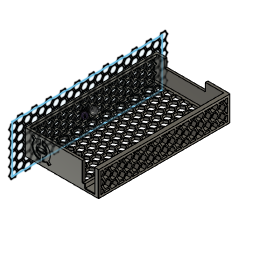
[a]BTT_MMB_case_top (Autodesk Fusion 360 design; units mm, degrees)
Autodesk Fusion 360 part; units mm, degrees
note: some values were not read from the file. Chosen so that the rebuilt part matches the saved one: which face or edge a step refers to. Set by a fixed rule: which sketch regions a step uses.
(part 1 of 3)
sketch "Top" plane through (0, 0, 0) normal (0, 0, 1) x (1, 0, 0)
  line L0 (8.6, 62.3) -> (62.6, 62.3) construction
  line L1 (62.6, 62.3) -> (62.6, -62.3) construction
  line L2 (62.6, -62.3) -> (8.6, -62.3) construction
  line L3 (8.6, -62.3) -> (8.6, 62.3) construction
  line L4 (8.6, 0) -> (0, 0) construction
  line L5 (62.8, -62.5) -> (8.4, -62.5)
  line L6 (8.4, -62.5) -> (8.4, 62.5)
  line L7 (8.4, 62.5) -> (62.8, 62.5)
  line L8 (62.8, 62.5) -> (62.8, -62.5)
  line L9 (6, -64.9) -> (6, 64.9)
  line L10 (6, 64.9) -> (65.2, 64.9)
  line L11 (65.2, 64.9) -> (65.2, -64.9)
  line L12 (65.2, -64.9) -> (6, -64.9)
  line L13 (8.6, 62.3) -> (13.6, 62.3) construction
  line L14 (13.6, 62.3) -> (13.6, 59.3) construction
  line L15 (13.6, 59.3) -> (8.6, 59.3) construction
  line L16 (8.6, 59.3) -> (8.6, 62.3) construction
  circle A0 centre (13.6, 59.3) radius 1.75
  circle A1 centre (13.6, 59.3) radius 5
  line L17 (13.6, 54.3) -> (8.4, 54.3)
  line L18 (18.6, 59.3) -> (18.6, 62.5)
  line L19 (35.6, 62.3) -> (35.6, 51.9797) construction
  circle A2 centre (57.6, 59.3) radius 5
  circle A3 centre (57.6, 59.3) radius 1.75
  line L20 (57.6, 54.3) -> (62.8, 54.3)
  line L21 (52.6, 59.3) -> (52.6, 62.5)
  line L22 (20, 0) -> (2.5, 0)
  circle A4 centre (13.6, -59.3) radius 5
  line L23 (18.6, -59.3) -> (18.6, -62.5)
  circle A5 centre (13.6, -59.3) radius 1.75
  line L24 (13.6, -54.3) -> (8.4, -54.3)
  circle A6 centre (57.6, -59.3) radius 1.75
  line L25 (57.6, -54.3) -> (62.8, -54.3)
  line L26 (52.6, -59.3) -> (52.6, -62.5)
  circle A7 centre (57.6, -59.3) radius 5
  line L27 (65.2, -64.9) -> (78.5, -64.9)
  line L28 (78.5, -64.9) -> (78.5, 64.9)
  line L29 (78.5, 64.9) -> (65.2, 64.9)
  line L30 (65.2, 64.9) -> (65.2, -64.9)
  line L31 (78.5, -64.9) -> (74.5, -64.9)
  line L32 (74.5, -64.9) -> (74.5, 64.9)
  line L33 (74.5, 64.9) -> (78.5, 64.9)
  line L34 (78.5, 64.9) -> (78.5, -64.9)
  line L35 (78.5, 64.9) -> (62.8, 64.9)
  line L36 (62.8, 64.9) -> (62.8, 62.5)
  line L37 (62.8, 62.5) -> (78.5, 62.5)
  line L38 (78.5, 62.5) -> (78.5, 64.9)
  line L39 (62.8, -62.5) -> (62.8, -64.9)
  line L40 (13.6, -54.3) -> (13.6, 54.3)
  line L41 (57.6, 54.3) -> (57.6, -54.3)
  line L42 (18.6, 62.5) -> (18.6, 64.9)
  line L43 (52.6, 62.5) -> (52.6, 64.9)
  circle A8 centre (13.6, 59.3) radius 2.95
  circle A9 centre (57.6, 59.3) radius 2.95
  circle A10 centre (57.6, -59.3) radius 2.95
  circle A11 centre (13.6, -59.3) radius 2.95
  line L44 (13.6, -54.3) -> (13.6, -62.5)
  line L45 (13.6, 54.3) -> (13.6, 62.5)
  line L46 (57.6, 54.3) -> (57.6, 62.5)
  line L47 (57.6, -54.3) -> (57.6, -62.5)
  line L48 (8.6, 60.1) -> (62.6, 60.1)
  line L49 (62.6, -60.1) -> (8.6, -60.1)
  line L50 (62.6, -60.1) -> (63.1136, -60.1)
  line L51 (8.6, -60.1) -> (8.2021, -60.1)
  line L52 (8.6, 60.1) -> (8.1648, 60.1)
  line L53 (62.6, 60.1) -> (63.3075, 60.1)
  line L54 (56.5, 64.9) -> (16.5, 64.9)
  line L55 (16.5, 64.9) -> (16.5, 54.9)
  line L56 (16.5, 54.9) -> (56.5, 54.9)
  line L57 (56.5, 54.9) -> (56.5, 64.9)
  line L58 (78.5, 64.9) -> (16.5, 64.9)
  point P0 (13.6, -59.3)
  dimension "d1" = 54
  dimension "d2" = 124.6
  dimension "d3" = 8.6
  dimension "d4" = -0.2
  dimension "d5" = -2.6
  dimension "d6" = 5
  dimension "d7" = 3
  dimension "d8" = 3.5
  dimension "d9" = 10
  dimension "d10" = 13.3
  dimension "d12" = 4
  dimension "d41" = 5.9
  dimension "d42" = 5.9
  dimension "d43" = 5.9
  dimension "d44" = 5.9
  dimension "d97" = 2.2
  dimension "d98" = 2.2
  dimension "d99" = 40
  dimension "d100" = 10
  dimension "d101" = 62
  dimension "d103" = 129.8
  constraint horizontal L0
  constraint vertical L1
  constraint horizontal L2
  constraint vertical L3
  constraint midpoint L3 L4.start
  constraint coincident L4.end origin
  constraint horizontal L4
  constraint horizontal L13
  constraint vertical L14
  constraint horizontal L15
  constraint vertical L16
  constraint coincident L14.end L15.start
  constraint concentric A0 A1
  constraint coincident A1 L17.start
  constraint coincident L6 L17.end
  constraint tangent A1 L17
  constraint perpendicular L6 L17
  constraint coincident A1 L18.start
  constraint coincident L7 L18.end
  constraint tangent A1 L18
  constraint perpendicular L7 L18
  constraint midpoint L0 L19.start
  constraint perpendicular L0 L19
  constraint symmetric A0 L19 A3
  constraint symmetric A1 L19 A2
  constraint symmetric L17.start L19 L20.start
  constraint symmetric L17.end L19 L20.end
  constraint symmetric L18.start L19 L21.start
  constraint symmetric L18.end L19 L21.end
  constraint symmetric L14.end L22 P0
  constraint symmetric A0 L22 A5
  constraint symmetric A1 L22 A4
  constraint symmetric L17.start L22 L24.start
  constraint symmetric L17.end L22 L24.end
  constraint symmetric L18.start L22 L23.start
  constraint symmetric L18.end L22 L23.end
  constraint symmetric L20.start L22 L25.start
  constraint symmetric A2 L22 A7
  constraint symmetric A3 L22 A6
  constraint symmetric L20.end L22 L25.end
  constraint symmetric L21.start L22 L26.start
  constraint symmetric L21.end L22 L26.end
  constraint horizontal L27
  constraint vertical L28
  constraint horizontal L29
  constraint vertical L30
  constraint horizontal L31
  constraint vertical L32
  constraint horizontal L33
  constraint vertical L34
  constraint coincident L29 L32.end
  constraint horizontal L35
  constraint vertical L36
  constraint horizontal L37
  constraint vertical L38
  constraint coincident L12 L39.end
  constraint perpendicular L12 L39
  constraint coincident L10 L42.end
  constraint perpendicular L10 L42
  constraint coincident L10 L43.end
  constraint perpendicular L10 L43
  constraint concentric A2 A9
  constraint concentric A6 A10
  constraint coincident P0 A4.centre
  constraint coincident L5 L44.end
  constraint perpendicular L5 L44
  constraint coincident L7 L45.end
  constraint perpendicular L7 L45
  constraint coincident L7 L46.end
  constraint perpendicular L7 L46
  constraint coincident L5 L47.end
  constraint perpendicular L5 L47
  constraint perpendicular L1 L50
  constraint perpendicular L6 L51
  constraint perpendicular L6 L52
  constraint perpendicular L8 L53
  constraint horizontal L54
  constraint vertical L55
  constraint horizontal L56
  constraint vertical L57
  constraint perpendicular L43 L58
  measures "d1" distance of L0.start L0.end
  measures "d2" distance of L0.start L2.end
  measures "d3" distance of L4.start L4.end
  measures "d6" distance of L0.start L13.end
  measures "d7" distance of L0.start L15.end
  measures "d8" diameter of A0
  measures "d9" diameter of A1
  measures "d10" distance of L11.end L27.end
  measures "d12" distance of L27.end L31.end
  measures "d41" diameter of A8
  measures "d42" diameter of A9
  measures "d43" diameter of A10
  measures "d44" diameter of A11
  measures "d99" distance of L54.start L54.end
  measures "d100" distance of L54.start L56.end
  measures "d101" distance of L28.end L54.end
  measures "d103" distance of L27.end L28.end
extrude "Extrude1" add sketch "Top" along normal blind 2.5 contours L5 L6 L9 L12 L22 A4 A7 L39 | L5 L26 A7 L49 | L5 L23 L26 L49 | L5 A4 L23 L49 | L5 A7 A10 L47 L49 | L5 A7 | L5 A4 | L5 A4 A11 L44 L49 | L5 A7 A10 L47 L49 | L5 L8 A7 L49 L50 | L5 A4 A11 L44 L49 | L5 L6 A4 L49 L51 | A6 A10 L47 L49 | A6 A10 L47 L49 | L8 L11 L12 L30 L37 L39 | A5 A11 L44 L49 | A5 A11 L44 L49 | A6 L47 L49 | A6 L47 L49 | A5 L44 L49 | A5 L44 L49 | L11 L27 L30 L32 L37 | L6 L7 L9 L10 A1 L22 L55 | L10 L11 L30 L35 L36 L37 L58 | L11 L29 L30 L32 L35 L37 L58 | L27 L28 L31 L32 L34 L37 | L7 L8 A2 L48 L53 | L7 A2 A9 L46 L48 | L6 L7 A1 L48 L52 | L7 A1 A8 L45 L48 | L7 L10 A2 L36 L57 L58 | L28 L29 L32 L33 L34 L35 L37 L38 L58 | L7 A2 L57 | A3 A9 L46 L48 | L7 A2 L21 L48 | L7 A2 A9 L48 L57 | L7 L18 L21 L48 | A3 A9 L48 L57 | A3 L46 L48 L57 | A3 L46 L48 | L7 A1 L55 | A0 A8 L45 L48 | L7 L10 A1 L42 L54 L55 L58 | L7 A9 L46 L57 | L7 A2 L57 | L7 L10 A2 L43 L54 L57 L58 | A3 A9 L46 L57 | L7 L10 L42 L43 L54 L58 | L7 A1 L18 L48 | A3 L48 L57 | L7 A8 L45 L48 L55 | L7 A1 L55 | A0 A8 L45 L48 | A0 L45 L48 | L7 A1 L48 L55 | A0 L45 L48 picked at (59.849, -60.491) picked at (55.351, -60.491) picked at (15.849, -60.491) picked at (11.351, -60.491) picked at (57.6797, -60.7279) picked at (57.5203, -60.7279) picked at (13.6797, -60.7279) picked at (13.5203, -60.7279) picked at (59.849, 60.491) picked at (55.3319, 60.4563) picked at (56.9315, 60.3325) picked at (57.6797, 60.7279) picked at (11.351, 60.491) picked at (56.8289, 61.7259) picked at (56.3305, 60.3011) picked at (15.849, 60.491) picked at (13.5203, 60.7279) picked at (13.6797, 60.7279) makes body 1
extrude "Extrude2" add sketch "Top" along normal blind 25.05 separate body contours L5 L6 L9 L12 L22 A4 A7 L39 | L5 A7 | L5 A4 | L6 L7 L9 L10 A1 L22 L55 | L10 L11 L30 L35 L36 L37 L58 | L11 L29 L30 L32 L35 L37 L58 | L27 L28 L31 L32 L34 L37 | L7 L10 A2 L36 L57 L58 | L28 L29 L32 L33 L34 L35 L37 L38 L58 | L7 A2 L57 | L7 A1 L55 picked at (57.0926, 63.094) picked at (15.3203, 62.9199) makes body 2 at (6, -21.6333, 16.7) makes body 3 at (78.5, 21.6333, 16.7)
extrude "Extrude3" add sketch "Top" along normal blind 17 contours L7 A1 L55 | L7 L10 A1 L42 L54 L55 L58 | L7 A2 L57 | L7 L10 A2 L43 L54 L57 L58 | L7 L10 L42 L43 L54 L58 | L7 A1 L55 picked at (56.2909, 63.5566) bodies 1 2 3
extrude "Extrude4" add sketch "Top" along normal blind 6.4 contours L8 L11 L12 L30 L37 L39 bodies 1
sketch "Logo?" plane through (0, 0, 0) normal (0, 1, 0) x (1, 0, 0)
  line L0 (0, 0) -> (22, 0)
  line L1 (22, -13.2) -> (22, 0) construction
  line L2 (22, -13.2) -> (22, -15) construction
  line L3 (22, -13.2) -> (22, -11.4) construction
  line L4 (19.65, -15) -> (24.35, -15)
  line L5 (19.65, -11.4) -> (24.35, -11.4)
  circle A0 centre (19.6404, -13.2) radius 1.8
  circle A1 centre (24.3416, -13.2) radius 1.8
  line L6 (22, -11.4) -> (22, -15) construction
  circle A2 centre (22, -13.2) radius 5
  circle A3 centre (22, -13.2) radius 9
  line L7 (22, -13.2) -> (28.364, -6.836) construction
  line L8 (22, -13.2) -> (31, -13.2) construction
  line L9 (22, -13.2) -> (15.636, -19.564) construction
  line L10 (22, -13.2) -> (31, -13.2) construction
  line L11 (21, -15) -> (23, -15)
  line L12 (23, -15) -> (23, -23.0446)
  line L13 (21, -15) -> (21, -23.9495)
  line L14 (21, -11.4) -> (21, -3.5444)
  line L15 (23.2543, -11.4) -> (23.2543, -2.8723)
  line L16 (14.6814, -18.3972) -> (16.8028, -20.5186)
  line L17 (14.6814, -18.3972) -> (17.9289, -18.3972) construction
  line L18 (15.636, -19.564) -> (15.7421, -19.4579)
  line L19 (14.6814, -18.3972) -> (12.5601, -20.5186)
  line L20 (16.8028, -20.5186) -> (14.6814, -22.6399)
  line L21 (22, -13.2) -> (22.0813, -13.2813)
  line L22 (22, -13.2) -> (17.5038, -8.7038) construction
  line L23 (22, -13.2) -> (28.3586, -13.2) construction
  line L24 (27.1972, -5.8814) -> (29.3186, -3.7601)
  line L25 (29.3186, -8.0028) -> (31.4399, -5.8814)
  line L26 (12.5601, -20.5186) -> (14.6814, -22.6399)
  line L27 (29.3186, -3.7601) -> (31.4399, -5.8814)
  dimension "d21" = 22
  dimension "d22" = 13.2
  dimension "d24" = 1.8
  dimension "d25" = 4.7
  dimension "d26" = 4.7
  dimension "d27" = 10
  dimension "d28" = 18
  dimension "d29" = 45
  dimension "d30" = 135
  dimension "d31" = 2
  dimension "d32" = 45
  dimension "d33" = 3
  dimension "d34" = 0.15
  dimension "d35" = 3
  dimension "d37" = 135
  constraint coincident L0.start origin
  constraint horizontal L0
  constraint perpendicular L0 L1
  constraint perpendicular L2 L4
  constraint perpendicular L1 L5
  constraint midpoint L2.end L4
  constraint midpoint L3.end L5
  constraint coincident L5.start A0
  constraint coincident L4.start A0
  constraint coincident L5.end A1
  constraint coincident L4.end A1
  constraint coincident L1.start L2.start
  constraint concentric A2 A3
  constraint horizontal L8
  constraint coincident A3 L7.end
  constraint horizontal L10
  constraint coincident A3 L9.end
  constraint perpendicular L2 L11
  constraint midpoint L2.end L11
  constraint perpendicular L4 L12
  constraint perpendicular L4 L13
  constraint coincident L5 L14.start
  constraint perpendicular L5 L14
  constraint coincident L5 L15.start
  constraint perpendicular L5 L15
  constraint vertical L13
  constraint horizontal L17
  constraint parallel L9 L18
  constraint midpoint L16 L18.end
  constraint perpendicular L16 L19
  constraint perpendicular L16 L20
  constraint perpendicular L9 L21
  constraint horizontal L23
  constraint symmetric L16.start L22 L24.start
  constraint symmetric L16.end L22 L25.start
  constraint symmetric L19.end L22 L24.end
  constraint symmetric L20.end L22 L25.end
  constraint perpendicular L20 L26
  measures "d21" distance of L0.start L0.end
  measures "d22" distance of L0.end L1.start
  measures "d24" distance of L1.start L3.end
  measures "d25" distance of L4.start L4.end
  measures "d26" distance of L5.start L5.end
  measures "d27" diameter of A2
  measures "d28" diameter of A3
  measures "d29" angle of L7 L8
  measures "d30" angle of L9 L10
  measures "d31" distance of L11.start L11.end
  measures "d32" angle of L16 L17
  measures "d33" distance of L16.start L16.end
  measures "d34" distance of L9.end L18.end
  measures "d35" distance of L16.start L19.end
  measures "d37" angle of L22 L23
extrude "Extrude5" cut sketch "Logo?" along normal blind 0.8 from surface at -64.9 contours L4 L5 A0 A1 L11 | A0 | A2 A3 L13 L14 L16 L19 L20 | A2 A3 L12 L15 | A3 L19 L20 L26 | A3 L16 L18 L20 | A3 L16 L18 L19 | A3 L24 L25 L27 bodies 1
extrude "Extrude6" [suppressed]
sketch "Top Hex" plane through (0, 0, 0) normal (0, 0, 1) x (1, 0, 0)
  line L0 (0, 0) -> (1, 0) construction
  line L1 (1, 0) -> (1, 2) construction
  line L2 (1, 2) -> (0, 2) construction
  line L3 (0, 2) -> (0, 0) construction
  line L4 (4.3758, 3.949) -> (1, 5.8981)
  line L5 (1, 5.8981) -> (-2.3758, 3.949)
  line L6 (-2.3758, 3.949) -> (-2.3758, 0.051)
  line L7 (-2.3758, 0.051) -> (1, -1.8981)
  line L8 (1, -1.8981) -> (4.3758, 0.051)
  line L9 (4.3758, 0.051) -> (4.3758, 3.949)
  line L10 (1, 2) -> (2.6879, 4.9236) construction
  line L11 (1, 2) -> (2.6879, -0.9236) construction
  line L12 (8.3546, 10.8404) -> (4.9788, 12.7895)
  line L13 (8.3546, 6.9424) -> (8.3546, 10.8404)
  line L14 (4.9788, 4.9933) -> (8.3546, 6.9424)
  line L15 (1.6029, 6.9424) -> (4.9788, 4.9933)
  line L16 (1.6029, 10.8404) -> (1.6029, 6.9424)
  line L17 (4.9788, 12.7895) -> (1.6029, 10.8404)
  line L18 (-26.5739, 91.794) -> (105.9394, 91.794)
  line L19 (105.9394, 91.794) -> (105.9394, -79.3105)
  line L20 (105.9394, -79.3105) -> (-26.5739, -79.3105)
  line L21 (-26.5739, -79.3105) -> (-26.5739, 91.794)
  line L22 (4.3758, 2) -> (5.5758, 2)
  line L23 (1.6029, -62.7776) -> (4.9788, -64.7267)
  line L24 (1.6029, -58.8796) -> (1.6029, -62.7776)
  line L25 (4.9788, -56.9305) -> (1.6029, -58.8796)
  line L26 (8.3546, -58.8796) -> (4.9788, -56.9305)
  line L27 (4.9788, -64.7267) -> (8.3546, -62.7776)
  line L28 (4.3758, -69.669) -> (4.3758, -65.771)
  line L29 (4.3758, -65.771) -> (1, -63.8219)
  line L30 (1, -63.8219) -> (-2.3758, -65.771)
  line L31 (-2.3758, -65.771) -> (-2.3758, -69.669)
  line L32 (-2.3758, -69.669) -> (1, -71.6181)
  line L33 (1, -71.6181) -> (4.3758, -69.669)
  line L34 (9.5604, -62.7776) -> (12.9363, -64.7267)
  line L35 (9.5604, -58.8796) -> (9.5604, -62.7776)
  line L36 (12.9363, -56.9305) -> (9.5604, -58.8796)
  line L37 (16.3121, -58.8796) -> (12.9363, -56.9305)
  line L38 (12.9363, -64.7267) -> (16.3121, -62.7776)
  line L39 (12.3333, -69.669) -> (12.3333, -65.771)
  line L40 (12.3333, -65.771) -> (8.9575, -63.8219)
  line L41 (8.9575, -63.8219) -> (5.5817, -65.771)
  line L42 (5.5817, -65.771) -> (5.5817, -69.669)
  line L43 (5.5817, -69.669) -> (8.9575, -71.6181)
  line L44 (8.9575, -71.6181) -> (12.3333, -69.669)
  line L45 (8.3546, -62.7776) -> (8.3546, -58.8796)
  line L46 (16.3121, -62.7776) -> (16.3121, -58.8796)
  line L47 (4.9788, 12.7895) -> (4.9788, 13.9895) construction
  line L48 (3.9166, 13.9895) -> (6.0409, 13.9895) construction
  line L49 (17.5179, -62.7776) -> (20.8938, -64.7267)
  line L50 (17.5179, -58.8796) -> (17.5179, -62.7776)
  line L51 (20.8938, -56.9305) -> (17.5179, -58.8796)
  line L52 (24.2696, -58.8796) -> (20.8938, -56.9305)
  line L53 (20.8938, -64.7267) -> (24.2696, -62.7776)
  line L54 (20.2908, -69.669) -> (20.2908, -65.771)
  line L55 (20.2908, -65.771) -> (16.915, -63.8219)
  line L56 (16.915, -63.8219) -> (13.5392, -65.771)
  line L57 (13.5392, -65.771) -> (13.5392, -69.669)
  line L58 (13.5392, -69.669) -> (16.915, -71.6181)
  line L59 (16.915, -71.6181) -> (20.2908, -69.669)
  line L60 (24.2696, -62.7776) -> (24.2696, -58.8796)
  line L61 (25.4754, -62.7776) -> (28.8513, -64.7267)
  line L62 (25.4754, -58.8796) -> (25.4754, -62.7776)
  line L63 (28.8513, -56.9305) -> (25.4754, -58.8796)
  line L64 (32.2271, -58.8796) -> (28.8513, -56.9305)
  line L65 (28.8513, -64.7267) -> (32.2271, -62.7776)
  line L66 (28.2483, -69.669) -> (28.2483, -65.771)
  line L67 (28.2483, -65.771) -> (24.8725, -63.8219)
  line L68 (24.8725, -63.8219) -> (21.4967, -65.771)
  line L69 (21.4967, -65.771) -> (21.4967, -69.669)
  line L70 (21.4967, -69.669) -> (24.8725, -71.6181)
  line L71 (24.8725, -71.6181) -> (28.2483, -69.669)
  line L72 (32.2271, -62.7776) -> (32.2271, -58.8796)
  line L73 (33.4329, -62.7776) -> (36.8088, -64.7267)
  line L74 (33.4329, -58.8796) -> (33.4329, -62.7776)
  line L75 (36.8088, -56.9305) -> (33.4329, -58.8796)
  line L76 (40.1846, -58.8796) -> (36.8088, -56.9305)
  line L77 (36.8088, -64.7267) -> (40.1846, -62.7776)
  line L78 (36.2058, -69.669) -> (36.2058, -65.771)
  line L79 (36.2058, -65.771) -> (32.83, -63.8219)
  line L80 (32.83, -63.8219) -> (29.4542, -65.771)
  line L81 (29.4542, -65.771) -> (29.4542, -69.669)
  line L82 (29.4542, -69.669) -> (32.83, -71.6181)
  line L83 (32.83, -71.6181) -> (36.2058, -69.669)
  line L84 (40.1846, -62.7776) -> (40.1846, -58.8796)
  line L85 (41.3904, -62.7776) -> (44.7663, -64.7267)
  line L86 (41.3904, -58.8796) -> (41.3904, -62.7776)
  line L87 (44.7663, -56.9305) -> (41.3904, -58.8796)
  line L88 (48.1421, -58.8796) -> (44.7663, -56.9305)
  line L89 (44.7663, -64.7267) -> (48.1421, -62.7776)
  line L90 (44.1633, -69.669) -> (44.1633, -65.771)
  line L91 (44.1633, -65.771) -> (40.7875, -63.8219)
  line L92 (40.7875, -63.8219) -> (37.4117, -65.771)
  line L93 (37.4117, -65.771) -> (37.4117, -69.669)
  line L94 (37.4117, -69.669) -> (40.7875, -71.6181)
  line L95 (40.7875, -71.6181) -> (44.1633, -69.669)
  line L96 (48.1421, -62.7776) -> (48.1421, -58.8796)
  line L97 (49.3479, -62.7776) -> (52.7238, -64.7267)
  line L98 (49.3479, -58.8796) -> (49.3479, -62.7776)
  line L99 (52.7238, -56.9305) -> (49.3479, -58.8796)
  line L100 (56.0996, -58.8796) -> (52.7238, -56.9305)
  line L101 (52.7238, -64.7267) -> (56.0996, -62.7776)
  line L102 (52.1208, -69.669) -> (52.1208, -65.771)
  line L103 (52.1208, -65.771) -> (48.745, -63.8219)
  line L104 (48.745, -63.8219) -> (45.3692, -65.771)
  line L105 (45.3692, -65.771) -> (45.3692, -69.669)
  line L106 (45.3692, -69.669) -> (48.745, -71.6181)
  line L107 (48.745, -71.6181) -> (52.1208, -69.669)
  line L108 (56.0996, -62.7776) -> (56.0996, -58.8796)
  line L109 (57.3054, -62.7776) -> (60.6813, -64.7267)
  line L110 (57.3054, -58.8796) -> (57.3054, -62.7776)
  line L111 (60.6813, -56.9305) -> (57.3054, -58.8796)
  line L112 (64.0571, -58.8796) -> (60.6813, -56.9305)
  line L113 (60.6813, -64.7267) -> (64.0571, -62.7776)
  line L114 (60.0783, -69.669) -> (60.0783, -65.771)
  line L115 (60.0783, -65.771) -> (56.7025, -63.8219)
  line L116 (56.7025, -63.8219) -> (53.3267, -65.771)
  line L117 (53.3267, -65.771) -> (53.3267, -69.669)
  line L118 (53.3267, -69.669) -> (56.7025, -71.6181)
  line L119 (56.7025, -71.6181) -> (60.0783, -69.669)
  line L120 (64.0571, -62.7776) -> (64.0571, -58.8796)
  line L121 (65.2629, -62.7776) -> (68.6388, -64.7267)
  line L122 (65.2629, -58.8796) -> (65.2629, -62.7776)
  line L123 (68.6388, -56.9305) -> (65.2629, -58.8796)
  line L124 (72.0146, -58.8796) -> (68.6388, -56.9305)
  line L125 (68.6388, -64.7267) -> (72.0146, -62.7776)
  line L126 (68.0358, -69.669) -> (68.0358, -65.771)
  line L127 (68.0358, -65.771) -> (64.66, -63.8219)
  line L128 (64.66, -63.8219) -> (61.2842, -65.771)
  line L129 (61.2842, -65.771) -> (61.2842, -69.669)
  line L130 (61.2842, -69.669) -> (64.66, -71.6181)
  line L131 (64.66, -71.6181) -> (68.0358, -69.669)
  line L132 (72.0146, -62.7776) -> (72.0146, -58.8796)
  line L133 (73.2204, -62.7776) -> (76.5963, -64.7267)
  line L134 (73.2204, -58.8796) -> (73.2204, -62.7776)
  line L135 (76.5963, -56.9305) -> (73.2204, -58.8796)
  line L136 (79.9721, -58.8796) -> (76.5963, -56.9305)
  line L137 (76.5963, -64.7267) -> (79.9721, -62.7776)
  line L138 (75.9933, -69.669) -> (75.9933, -65.771)
  line L139 (75.9933, -65.771) -> (72.6175, -63.8219)
  line L140 (72.6175, -63.8219) -> (69.2417, -65.771)
  line L141 (69.2417, -65.771) -> (69.2417, -69.669)
  line L142 (69.2417, -69.669) -> (72.6175, -71.6181)
  line L143 (72.6175, -71.6181) -> (75.9933, -69.669)
  line L144 (79.9721, -62.7776) -> (79.9721, -58.8796)
  line L145 (81.1779, -62.7776) -> (84.5538, -64.7267)
  line L146 (81.1779, -58.8796) -> (81.1779, -62.7776)
  line L147 (84.5538, -56.9305) -> (81.1779, -58.8796)
  line L148 (87.9296, -58.8796) -> (84.5538, -56.9305)
  line L149 (84.5538, -64.7267) -> (87.9296, -62.7776)
  line L150 (83.9508, -69.669) -> (83.9508, -65.771)
  line L151 (83.9508, -65.771) -> (80.575, -63.8219)
  line L152 (80.575, -63.8219) -> (77.1992, -65.771)
  line L153 (77.1992, -65.771) -> (77.1992, -69.669)
  line L154 (77.1992, -69.669) -> (80.575, -71.6181)
  line L155 (80.575, -71.6181) -> (83.9508, -69.669)
  line L156 (87.9296, -62.7776) -> (87.9296, -58.8796)
  line L157 (1.6029, -48.8336) -> (4.9788, -50.7827)
  line L158 (1.6029, -44.9356) -> (1.6029, -48.8336)
  line L159 (4.9788, -42.9865) -> (1.6029, -44.9356)
  line L160 (8.3546, -44.9356) -> (4.9788, -42.9865)
  line L161 (4.9788, -50.7827) -> (8.3546, -48.8336)
  line L162 (4.3758, -55.725) -> (4.3758, -51.827)
  line L163 (4.3758, -51.827) -> (1, -49.8779)
  line L164 (1, -49.8779) -> (-2.3758, -51.827)
  line L165 (-2.3758, -51.827) -> (-2.3758, -55.725)
  line L166 (-2.3758, -55.725) -> (1, -57.6741)
  line L167 (1, -57.6741) -> (4.3758, -55.725)
  line L168 (8.3546, -48.8336) -> (8.3546, -44.9356)
  line L169 (9.5604, -48.8336) -> (12.9363, -50.7827)
  line L170 (9.5604, -44.9356) -> (9.5604, -48.8336)
  line L171 (12.9363, -42.9865) -> (9.5604, -44.9356)
  line L172 (16.3121, -44.9356) -> (12.9363, -42.9865)
  line L173 (12.9363, -50.7827) -> (16.3121, -48.8336)
  line L174 (12.3333, -55.725) -> (12.3333, -51.827)
  line L175 (12.3333, -51.827) -> (8.9575, -49.8779)
  line L176 (8.9575, -49.8779) -> (5.5817, -51.827)
  line L177 (5.5817, -51.827) -> (5.5817, -55.725)
  line L178 (5.5817, -55.725) -> (8.9575, -57.6741)
  line L179 (8.9575, -57.6741) -> (12.3333, -55.725)
  line L180 (16.3121, -48.8336) -> (16.3121, -44.9356)
  line L181 (17.5179, -48.8336) -> (20.8938, -50.7827)
  line L182 (17.5179, -44.9356) -> (17.5179, -48.8336)
  line L183 (20.8938, -42.9865) -> (17.5179, -44.9356)
  line L184 (24.2696, -44.9356) -> (20.8938, -42.9865)
  line L185 (20.8938, -50.7827) -> (24.2696, -48.8336)
  line L186 (20.2908, -55.725) -> (20.2908, -51.827)
  line L187 (20.2908, -51.827) -> (16.915, -49.8779)
  line L188 (16.915, -49.8779) -> (13.5392, -51.827)
  line L189 (13.5392, -51.827) -> (13.5392, -55.725)
  line L190 (13.5392, -55.725) -> (16.915, -57.6741)
  line L191 (16.915, -57.6741) -> (20.2908, -55.725)
  line L192 (24.2696, -48.8336) -> (24.2696, -44.9356)
  line L193 (25.4754, -48.8336) -> (28.8513, -50.7827)
  line L194 (25.4754, -44.9356) -> (25.4754, -48.8336)
  line L195 (28.8513, -42.9865) -> (25.4754, -44.9356)
  line L196 (32.2271, -44.9356) -> (28.8513, -42.9865)
  line L197 (28.8513, -50.7827) -> (32.2271, -48.8336)
  line L198 (28.2483, -55.725) -> (28.2483, -51.827)
  line L199 (28.2483, -51.827) -> (24.8725, -49.8779)
  line L200 (24.8725, -49.8779) -> (21.4967, -51.827)
  line L201 (21.4967, -51.827) -> (21.4967, -55.725)
  line L202 (21.4967, -55.725) -> (24.8725, -57.6741)
  line L203 (24.8725, -57.6741) -> (28.2483, -55.725)
  line L204 (32.2271, -48.8336) -> (32.2271, -44.9356)
  line L205 (33.4329, -48.8336) -> (36.8088, -50.7827)
  line L206 (33.4329, -44.9356) -> (33.4329, -48.8336)
  line L207 (36.8088, -42.9865) -> (33.4329, -44.9356)
  line L208 (40.1846, -44.9356) -> (36.8088, -42.9865)
  line L209 (36.8088, -50.7827) -> (40.1846, -48.8336)
  line L210 (36.2058, -55.725) -> (36.2058, -51.827)
  line L211 (36.2058, -51.827) -> (32.83, -49.8779)
  line L212 (32.83, -49.8779) -> (29.4542, -51.827)
  line L213 (29.4542, -51.827) -> (29.4542, -55.725)
  line L214 (29.4542, -55.725) -> (32.83, -57.6741)
  line L215 (32.83, -57.6741) -> (36.2058, -55.725)
  line L216 (40.1846, -48.8336) -> (40.1846, -44.9356)
  line L217 (41.3904, -48.8336) -> (44.7663, -50.7827)
  line L218 (41.3904, -44.9356) -> (41.3904, -48.8336)
  line L219 (44.7663, -42.9865) -> (41.3904, -44.9356)
  line L220 (48.1421, -44.9356) -> (44.7663, -42.9865)
  line L221 (44.7663, -50.7827) -> (48.1421, -48.8336)
  line L222 (44.1633, -55.725) -> (44.1633, -51.827)
  line L223 (44.1633, -51.827) -> (40.7875, -49.8779)
  line L224 (40.7875, -49.8779) -> (37.4117, -51.827)
  line L225 (37.4117, -51.827) -> (37.4117, -55.725)
  line L226 (37.4117, -55.725) -> (40.7875, -57.6741)
  line L227 (40.7875, -57.6741) -> (44.1633, -55.725)
  line L228 (48.1421, -48.8336) -> (48.1421, -44.9356)
  line L229 (49.3479, -48.8336) -> (52.7238, -50.7827)
  line L230 (49.3479, -44.9356) -> (49.3479, -48.8336)
  line L231 (52.7238, -42.9865) -> (49.3479, -44.9356)
  line L232 (56.0996, -44.9356) -> (52.7238, -42.9865)
  line L233 (52.7238, -50.7827) -> (56.0996, -48.8336)
  line L234 (52.1208, -55.725) -> (52.1208, -51.827)
  line L235 (52.1208, -51.827) -> (48.745, -49.8779)
  line L236 (48.745, -49.8779) -> (45.3692, -51.827)
  line L237 (45.3692, -51.827) -> (45.3692, -55.725)
  line L238 (45.3692, -55.725) -> (48.745, -57.6741)
  line L239 (48.745, -57.6741) -> (52.1208, -55.725)
  line L240 (56.0996, -48.8336) -> (56.0996, -44.9356)
  line L241 (57.3054, -48.8336) -> (60.6813, -50.7827)
  line L242 (57.3054, -44.9356) -> (57.3054, -48.8336)
  line L243 (60.6813, -42.9865) -> (57.3054, -44.9356)
  line L244 (64.0571, -44.9356) -> (60.6813, -42.9865)
  line L245 (60.6813, -50.7827) -> (64.0571, -48.8336)
  line L246 (60.0783, -55.725) -> (60.0783, -51.827)
  line L247 (60.0783, -51.827) -> (56.7025, -49.8779)
  line L248 (56.7025, -49.8779) -> (53.3267, -51.827)
  line L249 (53.3267, -51.827) -> (53.3267, -55.725)
  line L250 (53.3267, -55.725) -> (56.7025, -57.6741)
  line L251 (56.7025, -57.6741) -> (60.0783, -55.725)
  line L252 (64.0571, -48.8336) -> (64.0571, -44.9356)
  line L253 (65.2629, -48.8336) -> (68.6388, -50.7827)
  line L254 (65.2629, -44.9356) -> (65.2629, -48.8336)
  line L255 (68.6388, -42.9865) -> (65.2629, -44.9356)
  line L256 (72.0146, -44.9356) -> (68.6388, -42.9865)
  line L257 (68.6388, -50.7827) -> (72.0146, -48.8336)
  line L258 (68.0358, -55.725) -> (68.0358, -51.827)
  line L259 (68.0358, -51.827) -> (64.66, -49.8779)
  line L260 (64.66, -49.8779) -> (61.2842, -51.827)
  line L261 (61.2842, -51.827) -> (61.2842, -55.725)
  line L262 (61.2842, -55.725) -> (64.66, -57.6741)
  line L263 (64.66, -57.6741) -> (68.0358, -55.725)
  line L264 (72.0146, -48.8336) -> (72.0146, -44.9356)
  line L265 (73.2204, -48.8336) -> (76.5963, -50.7827)
  line L266 (73.2204, -44.9356) -> (73.2204, -48.8336)
  line L267 (76.5963, -42.9865) -> (73.2204, -44.9356)
  line L268 (79.9721, -44.9356) -> (76.5963, -42.9865)
  line L269 (76.5963, -50.7827) -> (79.9721, -48.8336)
  line L270 (75.9933, -55.725) -> (75.9933, -51.827)
  line L271 (75.9933, -51.827) -> (72.6175, -49.8779)
  line L272 (72.6175, -49.8779) -> (69.2417, -51.827)
  line L273 (69.2417, -51.827) -> (69.2417, -55.725)
  line L274 (69.2417, -55.725) -> (72.6175, -57.6741)
  line L275 (72.6175, -57.6741) -> (75.9933, -55.725)
  line L276 (79.9721, -48.8336) -> (79.9721, -44.9356)
  line L277 (81.1779, -48.8336) -> (84.5538, -50.7827)
  line L278 (81.1779, -44.9356) -> (81.1779, -48.8336)
  line L279 (84.5538, -42.9865) -> (81.1779, -44.9356)
  line L280 (87.9296, -44.9356) -> (84.5538, -42.9865)
  line L281 (84.5538, -50.7827) -> (87.9296, -48.8336)
  line L282 (83.9508, -55.725) -> (83.9508, -51.827)
  line L283 (83.9508, -51.827) -> (80.575, -49.8779)
  line L284 (80.575, -49.8779) -> (77.1992, -51.827)
  line L285 (77.1992, -51.827) -> (77.1992, -55.725)
  line L286 (77.1992, -55.725) -> (80.575, -57.6741)
  line L287 (80.575, -57.6741) -> (83.9508, -55.725)
  line L288 (87.9296, -48.8336) -> (87.9296, -44.9356)
  line L289 (1.6029, -34.8896) -> (4.9788, -36.8387)
  line L290 (1.6029, -30.9916) -> (1.6029, -34.8896)
  line L291 (4.9788, -29.0425) -> (1.6029, -30.9916)
  line L292 (8.3546, -30.9916) -> (4.9788, -29.0425)
  line L293 (4.9788, -36.8387) -> (8.3546, -34.8896)
  line L294 (4.3758, -41.781) -> (4.3758, -37.883)
  line L295 (4.3758, -37.883) -> (1, -35.9339)
  line L296 (1, -35.9339) -> (-2.3758, -37.883)
  line L297 (-2.3758, -37.883) -> (-2.3758, -41.781)
  line L298 (-2.3758, -41.781) -> (1, -43.7301)
  line L299 (1, -43.7301) -> (4.3758, -41.781)
  line L300 (8.3546, -34.8896) -> (8.3546, -30.9916)
  line L301 (9.5604, -34.8896) -> (12.9363, -36.8387)
  line L302 (9.5604, -30.9916) -> (9.5604, -34.8896)
  line L303 (12.9363, -29.0425) -> (9.5604, -30.9916)
  line L304 (16.3121, -30.9916) -> (12.9363, -29.0425)
  line L305 (12.9363, -36.8387) -> (16.3121, -34.8896)
  line L306 (12.3333, -41.781) -> (12.3333, -37.883)
  line L307 (12.3333, -37.883) -> (8.9575, -35.9339)
  line L308 (8.9575, -35.9339) -> (5.5817, -37.883)
  line L309 (5.5817, -37.883) -> (5.5817, -41.781)
  line L310 (5.5817, -41.781) -> (8.9575, -43.7301)
  line L311 (8.9575, -43.7301) -> (12.3333, -41.781)
  line L312 (16.3121, -34.8896) -> (16.3121, -30.9916)
  line L313 (17.5179, -34.8896) -> (20.8938, -36.8387)
  line L314 (17.5179, -30.9916) -> (17.5179, -34.8896)
  line L315 (20.8938, -29.0425) -> (17.5179, -30.9916)
  line L316 (24.2696, -30.9916) -> (20.8938, -29.0425)
  line L317 (20.8938, -36.8387) -> (24.2696, -34.8896)
  line L318 (20.2908, -41.781) -> (20.2908, -37.883)
  line L319 (20.2908, -37.883) -> (16.915, -35.9339)
  line L320 (16.915, -35.9339) -> (13.5392, -37.883)
  line L321 (13.5392, -37.883) -> (13.5392, -41.781)
  line L322 (13.5392, -41.781) -> (16.915, -43.7301)
  line L323 (16.915, -43.7301) -> (20.2908, -41.781)
  line L324 (24.2696, -34.8896) -> (24.2696, -30.9916)
  line L325 (25.4754, -34.8896) -> (28.8513, -36.8387)
  line L326 (25.4754, -30.9916) -> (25.4754, -34.8896)
  line L327 (28.8513, -29.0425) -> (25.4754, -30.9916)
  line L328 (32.2271, -30.9916) -> (28.8513, -29.0425)
  line L329 (28.8513, -36.8387) -> (32.2271, -34.8896)
  line L330 (28.2483, -41.781) -> (28.2483, -37.883)
  line L331 (28.2483, -37.883) -> (24.8725, -35.9339)
  line L332 (24.8725, -35.9339) -> (21.4967, -37.883)
  line L333 (21.4967, -37.883) -> (21.4967, -41.781)
  line L334 (21.4967, -41.781) -> (24.8725, -43.7301)
  line L335 (24.8725, -43.7301) -> (28.2483, -41.781)
  line L336 (32.2271, -34.8896) -> (32.2271, -30.9916)
  line L337 (33.4329, -34.8896) -> (36.8088, -36.8387)
  line L338 (33.4329, -30.9916) -> (33.4329, -34.8896)
  line L339 (36.8088, -29.0425) -> (33.4329, -30.9916)
  line L340 (40.1846, -30.9916) -> (36.8088, -29.0425)
  line L341 (36.8088, -36.8387) -> (40.1846, -34.8896)
  line L342 (36.2058, -41.781) -> (36.2058, -37.883)
  line L343 (36.2058, -37.883) -> (32.83, -35.9339)
  line L344 (32.83, -35.9339) -> (29.4542, -37.883)
  line L345 (29.4542, -37.883) -> (29.4542, -41.781)
  line L346 (29.4542, -41.781) -> (32.83, -43.7301)
  line L347 (32.83, -43.7301) -> (36.2058, -41.781)
  line L348 (40.1846, -34.8896) -> (40.1846, -30.9916)
  line L349 (41.3904, -34.8896) -> (44.7663, -36.8387)
  line L350 (41.3904, -30.9916) -> (41.3904, -34.8896)
  line L351 (44.7663, -29.0425) -> (41.3904, -30.9916)
  line L352 (48.1421, -30.9916) -> (44.7663, -29.0425)
  line L353 (44.7663, -36.8387) -> (48.1421, -34.8896)
  line L354 (44.1633, -41.781) -> (44.1633, -37.883)
  line L355 (44.1633, -37.883) -> (40.7875, -35.9339)
  line L356 (40.7875, -35.9339) -> (37.4117, -37.883)
  line L357 (37.4117, -37.883) -> (37.4117, -41.781)
  line L358 (37.4117, -41.781) -> (40.7875, -43.7301)
  line L359 (40.7875, -43.7301) -> (44.1633, -41.781)
  line L360 (48.1421, -34.8896) -> (48.1421, -30.9916)
  line L361 (49.3479, -34.8896) -> (52.7238, -36.8387)
  line L362 (49.3479, -30.9916) -> (49.3479, -34.8896)
  line L363 (52.7238, -29.0425) -> (49.3479, -30.9916)
  line L364 (56.0996, -30.9916) -> (52.7238, -29.0425)
  line L365 (52.7238, -36.8387) -> (56.0996, -34.8896)
  line L366 (52.1208, -41.781) -> (52.1208, -37.883)
  line L367 (52.1208, -37.883) -> (48.745, -35.9339)
  line L368 (48.745, -35.9339) -> (45.3692, -37.883)
  line L369 (45.3692, -37.883) -> (45.3692, -41.781)
  line L370 (45.3692, -41.781) -> (48.745, -43.7301)
  line L371 (48.745, -43.7301) -> (52.1208, -41.781)
  line L372 (56.0996, -34.8896) -> (56.0996, -30.9916)
  line L373 (57.3054, -34.8896) -> (60.6813, -36.8387)
  line L374 (57.3054, -30.9916) -> (57.3054, -34.8896)
  line L375 (60.6813, -29.0425) -> (57.3054, -30.9916)
  line L376 (64.0571, -30.9916) -> (60.6813, -29.0425)
  line L377 (60.6813, -36.8387) -> (64.0571, -34.8896)
  line L378 (60.0783, -41.781) -> (60.0783, -37.883)
  line L379 (60.0783, -37.883) -> (56.7025, -35.9339)
  line L380 (56.7025, -35.9339) -> (53.3267, -37.883)
  line L381 (53.3267, -37.883) -> (53.3267, -41.781)
  line L382 (53.3267, -41.781) -> (56.7025, -43.7301)
  line L383 (56.7025, -43.7301) -> (60.0783, -41.781)
  line L384 (64.0571, -34.8896) -> (64.0571, -30.9916)
  line L385 (65.2629, -34.8896) -> (68.6388, -36.8387)
  line L386 (65.2629, -30.9916) -> (65.2629, -34.8896)
  line L387 (68.6388, -29.0425) -> (65.2629, -30.9916)
  line L388 (72.0146, -30.9916) -> (68.6388, -29.0425)
  line L389 (68.6388, -36.8387) -> (72.0146, -34.8896)
  line L390 (68.0358, -41.781) -> (68.0358, -37.883)
  line L391 (68.0358, -37.883) -> (64.66, -35.9339)
  line L392 (64.66, -35.9339) -> (61.2842, -37.883)
  line L393 (61.2842, -37.883) -> (61.2842, -41.781)
  line L394 (61.2842, -41.781) -> (64.66, -43.7301)
  line L395 (64.66, -43.7301) -> (68.0358, -41.781)
  line L396 (72.0146, -34.8896) -> (72.0146, -30.9916)
  line L397 (73.2204, -34.8896) -> (76.5963, -36.8387)
  line L398 (73.2204, -30.9916) -> (73.2204, -34.8896)
  line L399 (76.5963, -29.0425) -> (73.2204, -30.9916)
  line L400 (79.9721, -30.9916) -> (76.5963, -29.0425)
  line L401 (76.5963, -36.8387) -> (79.9721, -34.8896)
  line L402 (75.9933, -41.781) -> (75.9933, -37.883)
  line L403 (75.9933, -37.883) -> (72.6175, -35.9339)
  line L404 (72.6175, -35.9339) -> (69.2417, -37.883)
  line L405 (69.2417, -37.883) -> (69.2417, -41.781)
  line L406 (69.2417, -41.781) -> (72.6175, -43.7301)
  line L407 (72.6175, -43.7301) -> (75.9933, -41.781)
  line L408 (79.9721, -34.8896) -> (79.9721, -30.9916)
  line L409 (81.1779, -34.8896) -> (84.5538, -36.8387)
  line L410 (81.1779, -30.9916) -> (81.1779, -34.8896)
  line L411 (84.5538, -29.0425) -> (81.1779, -30.9916)
  line L412 (87.9296, -30.9916) -> (84.5538, -29.0425)
  line L413 (84.5538, -36.8387) -> (87.9296, -34.8896)
  line L414 (83.9508, -41.781) -> (83.9508, -37.883)
  line L415 (83.9508, -37.883) -> (80.575, -35.9339)
  line L416 (80.575, -35.9339) -> (77.1992, -37.883)
  line L417 (77.1992, -37.883) -> (77.1992, -41.781)
  line L418 (77.1992, -41.781) -> (80.575, -43.7301)
  line L419 (80.575, -43.7301) -> (83.9508, -41.781)
  line L420 (87.9296, -34.8896) -> (87.9296, -30.9916)
  line L421 (1.6029, -20.9456) -> (4.9788, -22.8947)
  line L422 (1.6029, -17.0476) -> (1.6029, -20.9456)
  line L423 (4.9788, -15.0985) -> (1.6029, -17.0476)
  line L424 (8.3546, -17.0476) -> (4.9788, -15.0985)
  line L425 (4.9788, -22.8947) -> (8.3546, -20.9456)
  line L426 (4.3758, -27.837) -> (4.3758, -23.939)
  line L427 (4.3758, -23.939) -> (1, -21.9899)
  line L428 (1, -21.9899) -> (-2.3758, -23.939)
  line L429 (-2.3758, -23.939) -> (-2.3758, -27.837)
  line L430 (-2.3758, -27.837) -> (1, -29.7861)
  line L431 (1, -29.7861) -> (4.3758, -27.837)
  line L432 (8.3546, -20.9456) -> (8.3546, -17.0476)
  line L433 (9.5604, -20.9456) -> (12.9363, -22.8947)
  line L434 (9.5604, -17.0476) -> (9.5604, -20.9456)
  line L435 (12.9363, -15.0985) -> (9.5604, -17.0476)
  line L436 (16.3121, -17.0476) -> (12.9363, -15.0985)
  line L437 (12.9363, -22.8947) -> (16.3121, -20.9456)
  line L438 (12.3333, -27.837) -> (12.3333, -23.939)
  line L439 (12.3333, -23.939) -> (8.9575, -21.9899)
  line L440 (8.9575, -21.9899) -> (5.5817, -23.939)
  line L441 (5.5817, -23.939) -> (5.5817, -27.837)
  line L442 (5.5817, -27.837) -> (8.9575, -29.7861)
  line L443 (8.9575, -29.7861) -> (12.3333, -27.837)
  line L444 (16.3121, -20.9456) -> (16.3121, -17.0476)
  line L445 (17.5179, -20.9456) -> (20.8938, -22.8947)
  line L446 (17.5179, -17.0476) -> (17.5179, -20.9456)
  line L447 (20.8938, -15.0985) -> (17.5179, -17.0476)
  line L448 (24.2696, -17.0476) -> (20.8938, -15.0985)
  line L449 (20.8938, -22.8947) -> (24.2696, -20.9456)
  line L450 (20.2908, -27.837) -> (20.2908, -23.939)
  line L451 (20.2908, -23.939) -> (16.915, -21.9899)
  line L452 (16.915, -21.9899) -> (13.5392, -23.939)
  line L453 (13.5392, -23.939) -> (13.5392, -27.837)
  line L454 (13.5392, -27.837) -> (16.915, -29.7861)
  line L455 (16.915, -29.7861) -> (20.2908, -27.837)
  line L456 (24.2696, -20.9456) -> (24.2696, -17.0476)
  line L457 (25.4754, -20.9456) -> (28.8513, -22.8947)
  line L458 (25.4754, -17.0476) -> (25.4754, -20.9456)
  line L459 (28.8513, -15.0985) -> (25.4754, -17.0476)
  line L460 (32.2271, -17.0476) -> (28.8513, -15.0985)
  line L461 (28.8513, -22.8947) -> (32.2271, -20.9456)
  line L462 (28.2483, -27.837) -> (28.2483, -23.939)
  line L463 (28.2483, -23.939) -> (24.8725, -21.9899)
  line L464 (24.8725, -21.9899) -> (21.4967, -23.939)
  line L465 (21.4967, -23.939) -> (21.4967, -27.837)
  line L466 (21.4967, -27.837) -> (24.8725, -29.7861)
  line L467 (24.8725, -29.7861) -> (28.2483, -27.837)
  line L468 (32.2271, -20.9456) -> (32.2271, -17.0476)
  line L469 (33.4329, -20.9456) -> (36.8088, -22.8947)
  line L470 (33.4329, -17.0476) -> (33.4329, -20.9456)
  line L471 (36.8088, -15.0985) -> (33.4329, -17.0476)
  line L472 (40.1846, -17.0476) -> (36.8088, -15.0985)
  line L473 (36.8088, -22.8947) -> (40.1846, -20.9456)
  line L474 (36.2058, -27.837) -> (36.2058, -23.939)
  line L475 (36.2058, -23.939) -> (32.83, -21.9899)
  line L476 (32.83, -21.9899) -> (29.4542, -23.939)
  line L477 (29.4542, -23.939) -> (29.4542, -27.837)
  line L478 (29.4542, -27.837) -> (32.83, -29.7861)
  line L479 (32.83, -29.7861) -> (36.2058, -27.837)
  line L480 (40.1846, -20.9456) -> (40.1846, -17.0476)
  line L481 (41.3904, -20.9456) -> (44.7663, -22.8947)
  line L482 (41.3904, -17.0476) -> (41.3904, -20.9456)
  line L483 (44.7663, -15.0985) -> (41.3904, -17.0476)
  line L484 (48.1421, -17.0476) -> (44.7663, -15.0985)
  line L485 (44.7663, -22.8947) -> (48.1421, -20.9456)
  line L486 (44.1633, -27.837) -> (44.1633, -23.939)
  line L487 (44.1633, -23.939) -> (40.7875, -21.9899)
  line L488 (40.7875, -21.9899) -> (37.4117, -23.939)
  line L489 (37.4117, -23.939) -> (37.4117, -27.837)
  line L490 (37.4117, -27.837) -> (40.7875, -29.7861)
  line L491 (40.7875, -29.7861) -> (44.1633, -27.837)
  line L492 (48.1421, -20.9456) -> (48.1421, -17.0476)
  line L493 (49.3479, -20.9456) -> (52.7238, -22.8947)
  line L494 (49.3479, -17.0476) -> (49.3479, -20.9456)
  line L495 (52.7238, -15.0985) -> (49.3479, -17.0476)
  line L496 (56.0996, -17.0476) -> (52.7238, -15.0985)
  line L497 (52.7238, -22.8947) -> (56.0996, -20.9456)
  line L498 (52.1208, -27.837) -> (52.1208, -23.939)
  line L499 (52.1208, -23.939) -> (48.745, -21.9899)
  line L500 (48.745, -21.9899) -> (45.3692, -23.939)
  line L501 (45.3692, -23.939) -> (45.3692, -27.837)
  line L502 (45.3692, -27.837) -> (48.745, -29.7861)
  line L503 (48.745, -29.7861) -> (52.1208, -27.837)
  line L504 (56.0996, -20.9456) -> (56.0996, -17.0476)
  line L505 (57.3054, -20.9456) -> (60.6813, -22.8947)
  line L506 (57.3054, -17.0476) -> (57.3054, -20.9456)
  line L507 (60.6813, -15.0985) -> (57.3054, -17.0476)
  line L508 (64.0571, -17.0476) -> (60.6813, -15.0985)
  line L509 (60.6813, -22.8947) -> (64.0571, -20.9456)
  line L510 (60.0783, -27.837) -> (60.0783, -23.939)
  line L511 (60.0783, -23.939) -> (56.7025, -21.9899)
  line L512 (56.7025, -21.9899) -> (53.3267, -23.939)
  line L513 (53.3267, -23.939) -> (53.3267, -27.837)
  line L514 (53.3267, -27.837) -> (56.7025, -29.7861)
  line L515 (56.7025, -29.7861) -> (60.0783, -27.837)
  line L516 (64.0571, -20.9456) -> (64.0571, -17.0476)
  line L517 (65.2629, -20.9456) -> (68.6388, -22.8947)
  line L518 (65.2629, -17.0476) -> (65.2629, -20.9456)
  line L519 (68.6388, -15.0985) -> (65.2629, -17.0476)
  line L520 (72.0146, -17.0476) -> (68.6388, -15.0985)
  line L521 (68.6388, -22.8947) -> (72.0146, -20.9456)
  line L522 (68.0358, -27.837) -> (68.0358, -23.939)
  line L523 (68.0358, -23.939) -> (64.66, -21.9899)
  line L524 (64.66, -21.9899) -> (61.2842, -23.939)
  line L525 (61.2842, -23.939) -> (61.2842, -27.837)
  line L526 (61.2842, -27.837) -> (64.66, -29.7861)
  line L527 (64.66, -29.7861) -> (68.0358, -27.837)
  line L528 (72.0146, -20.9456) -> (72.0146, -17.0476)
  line L529 (73.2204, -20.9456) -> (76.5963, -22.8947)
  line L530 (73.2204, -17.0476) -> (73.2204, -20.9456)
  line L531 (76.5963, -15.0985) -> (73.2204, -17.0476)
  line L532 (79.9721, -17.0476) -> (76.5963, -15.0985)
  line L533 (76.5963, -22.8947) -> (79.9721, -20.9456)
  line L534 (75.9933, -27.837) -> (75.9933, -23.939)
  line L535 (75.9933, -23.939) -> (72.6175, -21.9899)
  line L536 (72.6175, -21.9899) -> (69.2417, -23.939)
  line L537 (69.2417, -23.939) -> (69.2417, -27.837)
  line L538 (69.2417, -27.837) -> (72.6175, -29.7861)
  line L539 (72.6175, -29.7861) -> (75.9933, -27.837)
  line L540 (79.9721, -20.9456) -> (79.9721, -17.0476)
  line L541 (81.1779, -20.9456) -> (84.5538, -22.8947)
  line L542 (81.1779, -17.0476) -> (81.1779, -20.9456)
  line L543 (84.5538, -15.0985) -> (81.1779, -17.0476)
  line L544 (87.9296, -17.0476) -> (84.5538, -15.0985)
  line L545 (84.5538, -22.8947) -> (87.9296, -20.9456)
  line L546 (83.9508, -27.837) -> (83.9508, -23.939)
  line L547 (83.9508, -23.939) -> (80.575, -21.9899)
  line L548 (80.575, -21.9899) -> (77.1992, -23.939)
  line L549 (77.1992, -23.939) -> (77.1992, -27.837)
  line L550 (77.1992, -27.837) -> (80.575, -29.7861)
  line L551 (80.575, -29.7861) -> (83.9508, -27.837)
  line L552 (87.9296, -20.9456) -> (87.9296, -17.0476)
  line L553 (1.6029, -7.0016) -> (4.9788, -8.9507)
  line L554 (1.6029, -3.1036) -> (1.6029, -7.0016)
  line L555 (4.9788, -1.1545) -> (1.6029, -3.1036)
  line L556 (8.3546, -3.1036) -> (4.9788, -1.1545)
  line L557 (4.9788, -8.9507) -> (8.3546, -7.0016)
  line L558 (4.3758, -13.893) -> (4.3758, -9.995)
  line L559 (4.3758, -9.995) -> (1, -8.0459)
  line L560 (1, -8.0459) -> (-2.3758, -9.995)
  line L561 (-2.3758, -9.995) -> (-2.3758, -13.893)
  line L562 (-2.3758, -13.893) -> (1, -15.8421)
  line L563 (1, -15.8421) -> (4.3758, -13.893)
  line L564 (8.3546, -7.0016) -> (8.3546, -3.1036)
  line L565 (9.5604, -7.0016) -> (12.9363, -8.9507)
  line L566 (9.5604, -3.1036) -> (9.5604, -7.0016)
  line L567 (12.9363, -1.1545) -> (9.5604, -3.1036)
  line L568 (16.3121, -3.1036) -> (12.9363, -1.1545)
  line L569 (12.9363, -8.9507) -> (16.3121, -7.0016)
  line L570 (12.3333, -13.893) -> (12.3333, -9.995)
  line L571 (12.3333, -9.995) -> (8.9575, -8.0459)
  line L572 (8.9575, -8.0459) -> (5.5817, -9.995)
  line L573 (5.5817, -9.995) -> (5.5817, -13.893)
  line L574 (5.5817, -13.893) -> (8.9575, -15.8421)
  line L575 (8.9575, -15.8421) -> (12.3333, -13.893)
  line L576 (16.3121, -7.0016) -> (16.3121, -3.1036)
  line L577 (17.5179, -7.0016) -> (20.8938, -8.9507)
  line L578 (17.5179, -3.1036) -> (17.5179, -7.0016)
  line L579 (20.8938, -1.1545) -> (17.5179, -3.1036)
  line L580 (24.2696, -3.1036) -> (20.8938, -1.1545)
  line L581 (20.8938, -8.9507) -> (24.2696, -7.0016)
  line L582 (20.2908, -13.893) -> (20.2908, -9.995)
  line L583 (20.2908, -9.995) -> (16.915, -8.0459)
  line L584 (16.915, -8.0459) -> (13.5392, -9.995)
  line L585 (13.5392, -9.995) -> (13.5392, -13.893)
  line L586 (13.5392, -13.893) -> (16.915, -15.8421)
  line L587 (16.915, -15.8421) -> (20.2908, -13.893)
  line L588 (24.2696, -7.0016) -> (24.2696, -3.1036)
  line L589 (25.4754, -7.0016) -> (28.8513, -8.9507)
  line L590 (25.4754, -3.1036) -> (25.4754, -7.0016)
  line L591 (28.8513, -1.1545) -> (25.4754, -3.1036)
  line L592 (32.2271, -3.1036) -> (28.8513, -1.1545)
  line L593 (28.8513, -8.9507) -> (32.2271, -7.0016)
  line L594 (28.2483, -13.893) -> (28.2483, -9.995)
  line L595 (28.2483, -9.995) -> (24.8725, -8.0459)
  line L596 (24.8725, -8.0459) -> (21.4967, -9.995)
  line L597 (21.4967, -9.995) -> (21.4967, -13.893)
  line L598 (21.4967, -13.893) -> (24.8725, -15.8421)
  line L599 (24.8725, -15.8421) -> (28.2483, -13.893)
  line L600 (32.2271, -7.0016) -> (32.2271, -3.1036)
  line L601 (33.4329, -7.0016) -> (36.8088, -8.9507)
  line L602 (33.4329, -3.1036) -> (33.4329, -7.0016)
  line L603 (36.8088, -1.1545) -> (33.4329, -3.1036)
  line L604 (40.1846, -3.1036) -> (36.8088, -1.1545)
  line L605 (36.8088, -8.9507) -> (40.1846, -7.0016)
  line L606 (36.2058, -13.893) -> (36.2058, -9.995)
  line L607 (36.2058, -9.995) -> (32.83, -8.0459)
  line L608 (32.83, -8.0459) -> (29.4542, -9.995)
  line L609 (29.4542, -9.995) -> (29.4542, -13.893)
  line L610 (29.4542, -13.893) -> (32.83, -15.8421)
  line L611 (32.83, -15.8421) -> (36.2058, -13.893)
  line L612 (40.1846, -7.0016) -> (40.1846, -3.1036)
  line L613 (41.3904, -7.0016) -> (44.7663, -8.9507)
  line L614 (41.3904, -3.1036) -> (41.3904, -7.0016)
  line L615 (44.7663, -1.1545) -> (41.3904, -3.1036)
  line L616 (48.1421, -3.1036) -> (44.7663, -1.1545)
  line L617 (44.7663, -8.9507) -> (48.1421, -7.0016)
  line L618 (44.1633, -13.893) -> (44.1633, -9.995)
  line L619 (44.1633, -9.995) -> (40.7875, -8.0459)
  line L620 (40.7875, -8.0459) -> (37.4117, -9.995)
  line L621 (37.4117, -9.995) -> (37.4117, -13.893)
  line L622 (37.4117, -13.893) -> (40.7875, -15.8421)
  line L623 (40.7875, -15.8421) -> (44.1633, -13.893)
  line L624 (48.1421, -7.0016) -> (48.1421, -3.1036)
  line L625 (49.3479, -7.0016) -> (52.7238, -8.9507)
  line L626 (49.3479, -3.1036) -> (49.3479, -7.0016)
  line L627 (52.7238, -1.1545) -> (49.3479, -3.1036)
  line L628 (56.0996, -3.1036) -> (52.7238, -1.1545)
  line L629 (52.7238, -8.9507) -> (56.0996, -7.0016)
  line L630 (52.1208, -13.893) -> (52.1208, -9.995)
  line L631 (52.1208, -9.995) -> (48.745, -8.0459)
  line L632 (48.745, -8.0459) -> (45.3692, -9.995)
  line L633 (45.3692, -9.995) -> (45.3692, -13.893)
  line L634 (45.3692, -13.893) -> (48.745, -15.8421)
  line L635 (48.745, -15.8421) -> (52.1208, -13.893)
  line L636 (56.0996, -7.0016) -> (56.0996, -3.1036)
  line L637 (57.3054, -7.0016) -> (60.6813, -8.9507)
  line L638 (57.3054, -3.1036) -> (57.3054, -7.0016)
  line L639 (60.6813, -1.1545) -> (57.3054, -3.1036)
  line L640 (64.0571, -3.1036) -> (60.6813, -1.1545)
  line L641 (60.6813, -8.9507) -> (64.0571, -7.0016)
  line L642 (60.0783, -13.893) -> (60.0783, -9.995)
  line L643 (60.0783, -9.995) -> (56.7025, -8.0459)
  line L644 (56.7025, -8.0459) -> (53.3267, -9.995)
  line L645 (53.3267, -9.995) -> (53.3267, -13.893)
  line L646 (53.3267, -13.893) -> (56.7025, -15.8421)
  line L647 (56.7025, -15.8421) -> (60.0783, -13.893)
  line L648 (64.0571, -7.0016) -> (64.0571, -3.1036)
  line L649 (65.2629, -7.0016) -> (68.6388, -8.9507)
  line L650 (65.2629, -3.1036) -> (65.2629, -7.0016)
  line L651 (68.6388, -1.1545) -> (65.2629, -3.1036)
  line L652 (72.0146, -3.1036) -> (68.6388, -1.1545)
  line L653 (68.6388, -8.9507) -> (72.0146, -7.0016)
  line L654 (68.0358, -13.893) -> (68.0358, -9.995)
  line L655 (68.0358, -9.995) -> (64.66, -8.0459)
  line L656 (64.66, -8.0459) -> (61.2842, -9.995)
  line L657 (61.2842, -9.995) -> (61.2842, -13.893)
  line L658 (61.2842, -13.893) -> (64.66, -15.8421)
  line L659 (64.66, -15.8421) -> (68.0358, -13.893)
  line L660 (72.0146, -7.0016) -> (72.0146, -3.1036)
  line L661 (73.2204, -7.0016) -> (76.5963, -8.9507)
  line L662 (73.2204, -3.1036) -> (73.2204, -7.0016)
  line L663 (76.5963, -1.1545) -> (73.2204, -3.1036)
  line L664 (79.9721, -3.1036) -> (76.5963, -1.1545)
  line L665 (76.5963, -8.9507) -> (79.9721, -7.0016)
  line L666 (75.9933, -13.893) -> (75.9933, -9.995)
  line L667 (75.9933, -9.995) -> (72.6175, -8.0459)
  line L668 (72.6175, -8.0459) -> (69.2417, -9.995)
  line L669 (69.2417, -9.995) -> (69.2417, -13.893)
  line L670 (69.2417, -13.893) -> (72.6175, -15.8421)
  line L671 (72.6175, -15.8421) -> (75.9933, -13.893)
  line L672 (79.9721, -7.0016) -> (79.9721, -3.1036)